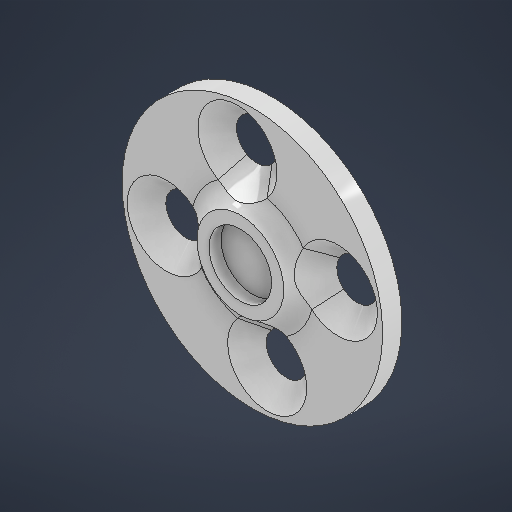
# Autodesk Inventor part: втулка для крепл
Saved by Autodesk Inventor 2025 (Build 290162000, 162)
## iProperties
Created: 2024-10-17
Part Number: втулка для крепл
Material: Пластик ПЭТ
Document SubType Name: Modeling
Designer: Phantom
Density: 1.541 g/cm^3
Appearance: Поликарбонат — прозрачный
Author: Phantom
Autodesk Inventor part; units mm, degrees
ref_plane "YZ Plane" through (0, 0, 0) normal (1, 0, 0) x (0, 1, 0)
ref_plane "XZ Plane" through (0, 0, 0) normal (0, 1, 0) x (-1, 0, 0)
ref_plane "XY Plane" through (0, 0, 0) normal (0, 0, 1) x (1, 0, 0)
sketch "Эскиз1" plane through (0, 0, 0) normal (0, 0, 1) x (1, 0, 0)
  circle A0 centre (0, 0) radius 3.25
  circle A1 centre (0, 0) radius 4.5
  dimension "d0" = 6.5
  dimension "d1" = 9
  constraints: 2 centre point, 2 coincident
  measures "d0" diameter of A0
  measures "d1" diameter of A1
extrude "Выдавливание1" add sketch "Эскиз1" along normal blind 5.25
sketch "Эскиз2" plane through (0, 0, 0) normal (0, 0, -1) x (-1, 0, 0)
  circle A0 centre (0, 0) radius 5.5
  dimension "d4" = 11
  constraints: 1 centre point, 1 coincident
  measures "d4" diameter of A0
loft "Лофт1" add profiles "Эскиз2" section 2 edges at (-4.5, 0, 5.25)
sketch "Эскиз4" plane through (0, 0, 0) normal (0, 0, -1) x (-1, 0, 0)
  circle A0 centre (0, 0) radius 3.25
  dimension "d10" = 6.5
  constraints: 1 centre point, 1 coincident
  measures "d10" diameter of A0
extrude "Выдавливание2" cut sketch "Эскиз4" against normal through all
sketch "Эскиз5" plane through (0, 0, 0) normal (0, 0, -1) x (-1, 0, 0)
  circle A0 centre (-8.8669, 1.5421) radius 2.1 projected
  circle A1 centre (-1.5421, -8.8669) radius 2.1 projected
  circle A2 centre (1.5421, 8.8669) radius 2.1 projected
  circle A3 centre (8.8669, -1.5421) radius 2.1 projected
  circle A4 centre (0, 0) radius 13.5
  circle A5 centre (0, 0) radius 3.25 projected
  dimension "d13" = 27
  constraints: 1 centre point, 1 coincident
  measures "d13" diameter of A4
extrude "Выдавливание3" add sketch "Эскиз5" against normal blind 4
fillet "Сопряжение1" radius 2 1 edges at (4.7381, 0, 4)
chamfer "Фаска1" distance 2 angle 45 4 edges at (0.5579, 8.8669, 4) (10.9669, 1.5421, 4) (-6.7669, -1.5421, 4) (3.6421, -8.8669, 4)
sketch "Эскиз6" plane through (0, 0, 0) normal (0, 0, -1) x (-1, 0, 0)
  circle A0 centre (0, 0) radius 13.5 projected
  circle A1 centre (8.8669, -1.5421) radius 2.1 projected
  circle A2 centre (1.5421, 8.8669) radius 2.1 projected
  circle A3 centre (-1.5421, -8.8669) radius 2.1 projected
  circle A4 centre (-8.8669, 1.5421) radius 2.1 projected
  circle A5 centre (0, 0) radius 3.25 projected
extrude "Выдавливание4" cut sketch "Эскиз6" against normal blind 2
sketch "Эскиз7" plane through (0, 0, 2) normal (0, 0, -1) x (-1, 0, 0)
  circle A0 centre (0, 0) radius 13.5 projected
  circle A1 centre (0, 0) radius 3.25 projected
  arc A2 (-7.0308, 2.5612) -> (-7.4827, -0.0371) centre (-8.8669, 1.5421) ccw projected
  arc A3 (-2.5612, -7.0308) -> (0.0371, -7.4827) centre (-1.5421, -8.8669) ccw projected
  arc A4 (2.5612, 7.0308) -> (-0.0371, 7.4827) centre (1.5421, 8.8669) ccw projected
  arc A5 (7.0308, -2.5612) -> (7.4827, 0.0371) centre (8.8669, -1.5421) ccw projected
  constraints: 4 other
extrude "Выдавливание5" add sketch "Эскиз7" against normal blind 2 contours A1
